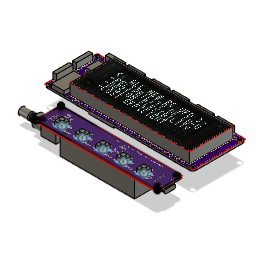
Overly Detailed Board Mockup (Autodesk Fusion 360 design; units mm, degrees)
Autodesk Fusion 360 part; units mm, degrees
sketch "Sketch1" plane through (0, 0, 0) normal (0, 1, 0) x (1, 0, 0)
  line L0 (0, 0) -> (24.384, 0)
  line L1 (24.384, 0) -> (24.384, 39.37)
  line L2 (24.384, 39.37) -> (0, 39.37)
  line L3 (0, 39.37) -> (0, 0)
  line L4 (7.1557, 6.35) -> (17.3157, 6.35)
  line L5 (17.3157, 6.35) -> (17.3157, 3.048)
  line L6 (17.3157, 3.048) -> (7.1557, 3.048)
  line L7 (7.1557, 3.048) -> (7.1557, 6.35)
  line L8 (7.1557, 6.35) -> (17.3157, 3.048) construction
  line L9 (17.3157, 6.35) -> (7.1557, 3.048) construction
  point P0 (12.2357, 4.699)
  dimension "d1" = 24.384
  dimension "d2" = 39.37
  dimension "d3" = 3.302
  dimension "d4" = 10.16
  dimension "d6" = 33.02
  constraint horizontal L0
  constraint vertical L1
  constraint horizontal L2
  constraint vertical L3
  constraint coincident L0.start L3.end
  constraint perpendicular L4 L5
  constraint parallel L4 L6
  constraint parallel L5 L7
  constraint horizontal L4
  constraint coincident L8 P0
  constraint coincident L9 P0
  measures "d1" distance of L0.start L0.end
  measures "d2" distance of L0.start L2.end
  measures "d3" distance of L4.end L5.end
  measures "d4" distance of L5.end L6.end
  measures "d6" distance of L2 L4
extrude "Extrude1" add sketch "Sketch1" along normal blind 1.905 contours L0 L1 L2 L3 | L4 L5 L6 L7 makes body 1
extrude "Extrude2" cut sketch "Sketch1" along normal through all contours L4 L5 L6 L7 bodies 1
sketch "Sketch2" plane through (0, 0, 0) normal (0, -1, 0) x (1, 0, 0)
  line L0 (17.3157, -3.048) -> (17.3157, -6.35)
  line L1 (17.3157, -6.35) -> (7.1557, -6.35)
  line L2 (7.1557, -6.35) -> (7.1557, -3.048)
  line L3 (7.1557, -3.048) -> (17.3157, -3.048)
  line L4 (0, 0) -> (0, -39.37)
  line L5 (0, -39.37) -> (24.384, -39.37)
  line L6 (24.384, -39.37) -> (24.384, 0)
  line L7 (24.384, 0) -> (0, 0)
  line L8 (-3.683, -39.37) -> (-2.54, -19.9644)
  line L9 (-2.54, -19.9644) -> (-1.8129, -7.62)
  line L10 (26.924, -19.9644) -> (26.1969, -7.62)
  line L11 (28.067, -39.37) -> (26.924, -19.9644)
  line L12 (-1.8129, -7.62) -> (26.1969, -7.62)
  line L13 (28.067, -39.37) -> (-3.683, -39.37)
  dimension "d15" = 93.371
  dimension "d16" = 93.371
  dimension "d17" = 31.75
  dimension "d18" = 31.75
  constraint parallel L8 L9
  constraint parallel L10 L11
  constraint horizontal L12
  constraint perpendicular L4 L13
  measures "d15" angle of L11 L13
  measures "d16" angle of L8 L13
  measures "d17" horizontal distance of L8.start L11.start
  measures "d18" distance of L12 L13
extrude "Extrude3" add sketch "Sketch2" along normal blind 3.175 contours L4 L5 L6 L12 L13 | L4 L8 L9 L12 L13 | L6 L10 L11 L12 L13 bodies 1
sketch "Sketch3" plane through (0, 0, -39.37) normal (0, 0, -1) x (-1, 0, 0)
  line L0 (0, 0) -> (0, 1.905)
  line L1 (0, 1.905) -> (-24.384, 1.905)
  line L2 (-24.384, 1.905) -> (-24.384, 0)
  line L3 (-24.384, 0) -> (-28.067, 0)
  line L4 (-28.067, 0) -> (-28.067, -3.175)
  line L5 (-28.067, -3.175) -> (3.683, -3.175)
  line L6 (3.683, -3.175) -> (3.683, 0)
  line L7 (3.683, 0) -> (0, 0)
  line L8 (-24.384, 0) -> (-28.067, -0.762)
  line L9 (0, 0) -> (3.683, -0.762)
  dimension "d21" = 0.762
  dimension "d22" = 0.762
  constraint coincident L2.end L3.start
  constraint coincident L4 L8.end
  constraint coincident L0.start L7.end
  constraint coincident L6 L9.end
  measures "d21" distance of L3.end L8.end
  measures "d22" distance of L6.end L9.end
extrude "Extrude4" cut sketch "Sketch3" against normal through all contours L0 L1 L2 L4 L5 L6 L8 L9 keep common part bodies 1
sketch "Sketch4" plane through (24.384, 0, 0) normal (1, 0, 0) x (0, 0, -1)
  line L0 (0, 0) -> (7.62, 0)
  line L1 (7.62, 0) -> (39.37, 0)
  line L2 (39.37, 0) -> (39.37, 1.905)
  line L3 (39.37, 1.905) -> (0, 1.905)
  line L4 (0, 1.905) -> (0, 0)
  line L5 (0, 1.905) -> (3.048, 0)
  line L6 (3.048, 0) -> (0, 0)
  line L7 (0, 1.905) -> (0, 0)
  point P0 (3.048, 0)
  constraint coincident L3.end L4.start
  constraint coincident P0 L5.end
  constraint coincident L0.start L4.end
extrude "Extrude5" cut sketch "Sketch4" against normal through all contours L0 L4 L5 L6 L7 bodies 1
sketch "Sketch5" plane through (0, 0, 0) normal (0, 1, 0) x (1, 0, 0)
  line L0 (2.54, 0) -> (116.84, 0)
  line L1 (119.38, 2.54) -> (119.38, 40.132)
  line L2 (116.84, 42.672) -> (2.54, 42.672)
  line L3 (0, 40.132) -> (0, 2.54)
  arc A0 (2.54, 42.672) -> (0, 40.132) centre (2.54, 40.132) ccw
  arc A1 (0, 2.54) -> (2.54, 0) centre (2.54, 2.54) ccw
  arc A2 (116.84, 0) -> (119.38, 2.54) centre (116.84, 2.54) ccw
  arc A3 (119.38, 40.132) -> (116.84, 42.672) centre (116.84, 40.132) ccw
  circle A4 centre (2.54, 40.132) radius 1.4132
  circle A5 centre (116.84, 40.132) radius 1.4368
  circle A6 centre (116.8086, 2.6914) radius 1.4384
  circle A7 centre (2.54, 2.6919) radius 1.4095
  point P0 (119.38, 0)
  point P1 (0, 42.672)
  dimension "d25" = 42.672
  dimension "d26" = 119.38
  dimension "d27" = 2.54
  dimension "d28" = 2.54
  dimension "d29" = 2.54
  dimension "d30" = 2.54
  constraint horizontal L0
  constraint vertical L1
  constraint horizontal L2
  constraint vertical L3
  constraint coincident P1 L2
  constraint coincident P1 L3
  constraint tangent L2 A0
  constraint tangent L3 A0
  constraint coincident origin L0
  constraint coincident origin L3
  constraint tangent L0 A1
  constraint tangent L3 A1
  constraint coincident P0 L1
  constraint coincident P0 L0
  constraint tangent L1 A2
  constraint tangent L0 A2
  constraint tangent L2 A3
  constraint tangent L1 A3
  constraint concentric A0 A4
  constraint concentric A3 A5
  measures "d25" distance of origin P1
  measures "d26" distance of origin P0
  measures "d27" radius of A0
  measures "d28" radius of A1
  measures "d29" radius of A2
  measures "d30" radius of A3
extrude "Extrude6" add sketch "Sketch5" against normal blind 1.6256 separate body makes body 2
sketch "Sketch6" plane through (0, 0, 0) normal (0, 1, 0) x (-1, 0, 0)
  circle A0 centre (-2.54, -2.6919) radius 1.4095
  circle A1 centre (-116.8086, -2.6914) radius 1.4384
  circle A2 centre (-2.54, -40.132) radius 1.4132
  circle A3 centre (-116.84, -40.132) radius 1.4368
  arc A4 (-119.38, -40.132) -> (-116.84, -42.672) centre (-116.84, -40.132) ccw
  line L0 (-116.84, -42.672) -> (-2.54, -42.672)
  arc A5 (-2.54, -42.672) -> (0, -40.132) centre (-2.54, -40.132) ccw
  line L1 (0, -40.132) -> (0, -2.54)
  arc A6 (0, -2.54) -> (-2.54, 0) centre (-2.54, -2.54) ccw
  line L2 (-2.54, 0) -> (-116.84, 0)
  arc A7 (-116.84, 0) -> (-119.38, -2.54) centre (-116.84, -2.54) ccw
  line L3 (-119.38, -2.54) -> (-119.38, -40.132)
  line L4 (-18.034, -2.667) -> (-113.9534, -2.667)
  line L5 (-113.9534, -2.667) -> (-113.9534, -37.5746)
  line L6 (-113.9534, -37.5746) -> (-18.034, -37.5746)
  line L7 (-18.034, -37.5746) -> (-18.034, -2.667)
  line L8 (-3.048, -6.858) -> (0, -6.858)
  line L9 (0, -6.858) -> (0, -20.066)
  line L10 (0, -20.066) -> (-3.048, -20.066)
  line L11 (-3.048, -20.066) -> (-3.048, -6.858)
  line L12 (-3.048, -22.7169) -> (0, -22.7169)
  line L13 (0, -22.7169) -> (0, -35.9458)
  line L14 (0, -35.9458) -> (-3.048, -35.9458)
  line L15 (-3.048, -35.9458) -> (-3.048, -22.7169)
  line L16 (-9.5782, -39.5447) -> (-22.7925, -39.5447)
  line L17 (-22.7925, -39.5447) -> (-22.7925, -42.672)
  line L18 (-22.7925, -42.672) -> (-9.5782, -42.672)
  line L19 (-9.5782, -42.672) -> (-9.5782, -39.5447)
  line L20 (-25.4303, -39.5447) -> (-38.6971, -39.5447)
  line L21 (-38.6971, -39.5447) -> (-38.6971, -42.672)
  line L22 (-38.6971, -42.672) -> (-25.4303, -42.672)
  line L23 (-25.4303, -42.672) -> (-25.4303, -39.5447)
  line L24 (-45.085, -39.624) -> (-58.3441, -39.624)
  line L25 (-58.3441, -39.624) -> (-58.3441, -42.672)
  line L26 (-58.3441, -42.672) -> (-45.085, -42.672)
  line L27 (-45.085, -42.672) -> (-45.085, -39.624)
  line L28 (-60.957, -39.5595) -> (-74.2397, -39.5595)
  line L29 (-74.2397, -39.5595) -> (-74.2397, -42.672)
  line L30 (-74.2397, -42.672) -> (-60.957, -42.672)
  line L31 (-60.957, -42.672) -> (-60.957, -39.5595)
  line L32 (-80.7977, -39.5595) -> (-94.107, -39.5595)
  line L33 (-94.107, -39.5595) -> (-94.107, -42.672)
  line L34 (-94.107, -42.672) -> (-80.7977, -42.672)
  line L35 (-80.7977, -42.672) -> (-80.7977, -39.5595)
  line L36 (-97.0058, -39.5595) -> (-110.2962, -39.5595)
  line L37 (-110.2962, -39.5595) -> (-110.2962, -42.672)
  line L38 (-110.2962, -42.672) -> (-97.0058, -42.672)
  line L39 (-97.0058, -42.672) -> (-97.0058, -39.5595)
  line L40 (-5.8246, -17.9754) -> (-15.8155, -17.9754)
  line L41 (-15.8155, -17.9754) -> (-15.8155, -0.0082)
  line L42 (-15.8155, -0.0082) -> (-5.8246, -0.0082)
  line L43 (-5.8246, -0.0082) -> (-5.8246, -17.9754)
  line L44 (-6.9981, -36.3389) -> (-17.116, -36.3389)
  line L45 (-17.116, -36.3389) -> (-17.116, -26.105)
  line L46 (-17.116, -26.105) -> (-6.9981, -26.105)
  line L47 (-6.9981, -26.105) -> (-6.9981, -36.3389)
  constraint horizontal L4
  constraint vertical L5
  constraint horizontal L6
  constraint vertical L7
  constraint horizontal L8
  constraint vertical L9
  constraint horizontal L10
  constraint vertical L11
  constraint coincident L1 L9.end
  constraint horizontal L12
  constraint vertical L13
  constraint horizontal L14
  constraint vertical L15
  constraint coincident L1 L13.end
  constraint horizontal L16
  constraint vertical L17
  constraint horizontal L18
  constraint vertical L19
  constraint coincident L0 L17.end
  constraint horizontal L20
  constraint vertical L21
  constraint horizontal L22
  constraint vertical L23
  constraint coincident L0 L21.end
  constraint horizontal L24
  constraint vertical L25
  constraint horizontal L26
  constraint vertical L27
  constraint coincident L0 L25.end
  constraint horizontal L28
  constraint vertical L29
  constraint horizontal L30
  constraint vertical L31
  constraint coincident L0 L29.end
  constraint horizontal L32
  constraint vertical L33
  constraint horizontal L34
  constraint vertical L35
  constraint coincident L0 L33.end
  constraint horizontal L36
  constraint vertical L37
  constraint horizontal L38
  constraint vertical L39
  constraint coincident L0 L37.end
  constraint horizontal L40
  constraint vertical L41
  constraint horizontal L42
  constraint vertical L43
  constraint horizontal L44
  constraint vertical L45
  constraint horizontal L46
  constraint vertical L47
extrude "Extrude8" add sketch "Sketch6" along normal blind 8.5 separate body contours L4 L5 L6 L7 makes body 3
extrude "Extrude9" add sketch "Sketch6" along normal blind 5 separate body contours L0 L36 L37 L38 L39 | L0 L32 L33 L34 L35 | L1 L8 L9 L10 L11 | L0 L28 L29 L30 L31 | L1 L12 L13 L14 L15 | L0 L24 L25 L26 L27 | L0 L20 L21 L22 L23 | L0 L16 L17 L18 L19 makes body 4 at (65.3846, 1.6667, -39.5595) makes body 5 at (0, 1.6667, -15.6633) makes body 6 at (18.3877, 1.6667, -42.672) makes body 7 at (85.2341, 1.6667, -39.5595) makes body 8 at (49.5047, 1.6667, -39.624) makes body 9 at (0, 1.6667, -31.5362) makes body 10 at (29.8526, 1.6667, -39.5447) makes body 11 at (101.4359, 1.6667, -39.5595)
combine "Combine1" operation add target body 2 tool bodies 11 3 4 5 6 8 7 10 9
extrude "Extrude10" add sketch "Sketch6" along normal blind 3.2 contours L40 L41 L42 L43 bodies 2
extrude "Extrude11" add sketch "Sketch6" along normal blind 2.1 contours L44 L45 L46 L47 bodies 2
copy_body "Body->Comp1" bodies 2 removing the originals makes body 12 in component "Mainboard Mockup"
sketch "Sketch7" plane through (0, -1.6256, 0) normal (0, -1, 0) x (1, 0, 0)
  circle A0 centre (2.54, -2.6919) radius 1.4095
  circle A1 centre (116.8086, -2.6914) radius 1.4384
  circle A2 centre (2.54, -40.132) radius 1.4132
  circle A3 centre (116.84, -40.132) radius 1.4368
  arc A4 (116.84, -42.672) -> (119.38, -40.132) centre (116.84, -40.132) ccw
  line L0 (119.38, -40.132) -> (119.38, -2.54)
  arc A5 (119.38, -2.54) -> (116.84, 0) centre (116.84, -2.54) ccw
  line L1 (116.84, 0) -> (2.54, 0)
  arc A6 (2.54, 0) -> (0, -2.54) centre (2.54, -2.54) ccw
  line L2 (0, -2.54) -> (0, -40.132)
  arc A7 (0, -40.132) -> (2.54, -42.672) centre (2.54, -40.132) ccw
  line L3 (2.54, -42.672) -> (116.84, -42.672)
  line L4 (56.9773, -8.2444) -> (34.4218, -8.2444)
  line L5 (34.4218, -8.2444) -> (34.4218, -13.7635)
  line L6 (34.4218, -13.7635) -> (56.9773, -13.7635)
  line L7 (56.9773, -13.7635) -> (56.9773, -8.2444)
  line L8 (55.7007, -8.2444) -> (35.814, -8.2444)
  line L9 (35.814, -8.2444) -> (35.814, 0)
  line L10 (35.814, 0) -> (55.7007, 0)
  line L11 (55.7007, 0) -> (55.7007, -8.2444)
  line L12 (109.728, -3.302) -> (74.168, -3.302)
  line L13 (74.168, -3.302) -> (74.168, -1.778)
  line L14 (74.168, -1.778) -> (109.728, -1.778)
  line L15 (109.728, -1.778) -> (109.728, -3.302)
  line L16 (29.21, -3.302) -> (23.622, -3.302)
  line L17 (23.622, -3.302) -> (23.622, -1.778)
  line L18 (23.622, -1.778) -> (29.21, -1.778)
  line L19 (29.21, -1.778) -> (29.21, -3.302)
  circle A8 centre (103.2884, -11.0072) radius 4.825
  constraint horizontal L4
  constraint vertical L5
  constraint horizontal L6
  constraint vertical L7
  constraint horizontal L8
  constraint vertical L9
  constraint horizontal L10
  constraint vertical L11
  constraint coincident L1 L9.end
  constraint coincident L4 L8.start
  constraint horizontal L12
  constraint vertical L13
  constraint horizontal L14
  constraint vertical L15
  constraint horizontal L16
  constraint vertical L17
  constraint horizontal L18
  constraint vertical L19
extrude "Extrude1'" add sketch "Sketch7" along normal blind 1.905 contours L1 L4 L8 L9 L10 L11 | L12 L13 L14 L15 | L16 L17 L18 L19 bodies 12 in component "Mainboard Mockup"
extrude "Extrude2'" add sketch "Sketch7" along normal blind 2 contours L4 L5 L6 L7 L8 bodies 12 in component "Mainboard Mockup"
extrude "Extrude3'" add sketch "Sketch7" along normal blind 3 contours A8 bodies 12 in component "Mainboard Mockup"
extrude "Extrude4'" cut 1 faces at (49.0718, -3.5306, -5.4963) along direction (0, 1, 0) blind 0.635 on bodies 12 bodies 12 in component "Mainboard Mockup"
sketch "Sketch1 (2)" plane through (0, 0, 0) normal (0, 1, 0) x (1, 0, 0) in component "Control Board Mockup"
  line L0 (2.54, 0) -> (95.25, 0)
  line L1 (97.79, 2.54) -> (97.79, 17.78)
  line L2 (95.25, 20.32) -> (2.54, 20.32)
  line L3 (0, 17.78) -> (0, 2.54)
  arc A0 (2.54, 20.32) -> (0, 17.78) centre (2.54, 17.78) ccw
  arc A1 (0, 2.54) -> (2.54, 0) centre (2.54, 2.54) ccw
  arc A2 (97.79, 17.78) -> (95.25, 20.32) centre (95.25, 17.78) ccw
  arc A3 (95.25, 0) -> (97.79, 2.54) centre (95.25, 2.54) ccw
  line L4 (11.7174, 3.3756) -> (17.6784, 3.3756)
  line L5 (17.6784, 3.3756) -> (17.6784, 9.3472)
  line L6 (17.6784, 9.3472) -> (11.7174, 9.3472)
  line L7 (11.7174, 9.3472) -> (11.7174, 3.3756)
  circle A4 centre (14.732, 6.35) radius 1.7145
  circle A5 centre (31.1912, 6.35) radius 1.7145
  line L8 (28.1766, 9.3472) -> (28.1766, 3.3756)
  line L9 (34.1376, 9.3472) -> (28.1766, 9.3472)
  line L10 (28.1766, 3.3756) -> (34.1376, 3.3756)
  line L11 (34.1376, 3.3756) -> (34.1376, 9.3472)
  circle A6 centre (47.6504, 6.35) radius 1.7145
  line L12 (44.6358, 9.3472) -> (44.6358, 3.3756)
  line L13 (50.5968, 9.3472) -> (44.6358, 9.3472)
  line L14 (44.6358, 3.3756) -> (50.5968, 3.3756)
  line L15 (50.5968, 3.3756) -> (50.5968, 9.3472)
  circle A7 centre (64.1096, 6.35) radius 1.7145
  line L16 (61.095, 9.3472) -> (61.095, 3.3756)
  line L17 (67.056, 9.3472) -> (61.095, 9.3472)
  line L18 (61.095, 3.3756) -> (67.056, 3.3756)
  line L19 (67.056, 3.3756) -> (67.056, 9.3472)
  circle A8 centre (80.5688, 6.35) radius 1.7145
  line L20 (77.5542, 9.3472) -> (77.5542, 3.3756)
  line L21 (83.5152, 9.3472) -> (77.5542, 9.3472)
  line L22 (77.5542, 3.3756) -> (83.5152, 3.3756)
  line L23 (83.5152, 3.3756) -> (83.5152, 9.3472)
  point P0 (97.79, 0)
  point P1 (0, 20.32)
  dimension "d51" = 97.79
  dimension "d52" = 20.32
  dimension "d53" = 2.54
  dimension "d54" = 2.54
  dimension "d55" = 2.54
  dimension "d56" = 2.54
  dimension "d57" = 3.429
  dimension "d60" = 16.4592
  dimension "d61" = 0
  constraint horizontal L0
  constraint vertical L1
  constraint horizontal L2
  constraint vertical L3
  constraint coincident P1 L2
  constraint coincident P1 L3
  constraint tangent L2 A0
  constraint tangent L3 A0
  constraint coincident origin L0
  constraint coincident origin L3
  constraint tangent L0 A1
  constraint tangent L3 A1
  constraint tangent L2 A2
  constraint tangent L1 A2
  constraint coincident P0 L1
  constraint coincident P0 L0
  constraint tangent L1 A3
  constraint tangent L0 A3
  constraint horizontal L4
  constraint vertical L5
  constraint horizontal L6
  constraint vertical L7
  measures "d51" distance of origin P0
  measures "d52" distance of origin P1
  measures "d53" radius of A0
  measures "d54" radius of A1
  measures "d55" radius of A2
  measures "d56" radius of A3
  measures "d57" diameter of A4
extrude "Extrude1''" add sketch "Sketch1 (2)" against normal blind 1.6256 separate body contours L0 L1 L2 L3 A0 A1 A2 A3 | L4 L5 L6 L7 | A4 | A5 | L8 L9 L10 L11 | A6 | L12 L13 L14 L15 | A7 | L16 L17 L18 L19 | A8 | L20 L21 L22 L23 makes body 13 in component "Control Board Mockup"
extrude "Extrude2''" add sketch "Sketch1 (2)" along normal blind 3.81 contours L4 L5 L6 L7 | L8 L9 L10 L11 | L12 L13 L14 L15 | L16 L17 L18 L19 | L20 L21 L22 L23 bodies 13 in component "Control Board Mockup"
extrude "Extrude3''" add sketch "Sketch1 (2)" along normal blind 5.0038 contours A4 | A5 | A6 | A7 | A8 bodies 13 in component "Control Board Mockup"
sketch "Sketch2 (2)" plane through (0, -1.6256, 0) normal (0, -1, 0) x (1, 0, 0) in component "Control Board Mockup"
  arc A0 (97.79, -2.54) -> (95.25, 0) centre (95.25, -2.54) ccw
  line L0 (95.25, 0) -> (2.54, 0)
  arc A1 (2.54, 0) -> (0, -2.54) centre (2.54, -2.54) ccw
  line L1 (0, -2.54) -> (0, -17.78)
  arc A2 (0, -17.78) -> (2.54, -20.32) centre (2.54, -17.78) ccw
  line L2 (2.54, -20.32) -> (95.25, -20.32)
  arc A3 (95.25, -20.32) -> (97.79, -17.78) centre (95.25, -17.78) ccw
  line L3 (97.79, -17.78) -> (97.79, -2.54)
  line L4 (12.0798, -13.738) -> (0, -13.738)
  line L5 (0, -13.738) -> (0, -4.064)
  line L6 (0, -4.064) -> (12.0798, -4.064)
  line L7 (12.0798, -4.064) -> (12.0798, -13.738)
  line L8 (18.3553, -1.1964) -> (78.1042, -1.1964)
  line L9 (78.1042, -1.1964) -> (78.1042, -16.6847)
  line L10 (78.1042, -16.6847) -> (18.3553, -16.6847)
  line L11 (18.3553, -16.6847) -> (18.3553, -1.1964)
  line L12 (88.2501, -13.6825) -> (98.7501, -13.6825)
  line L13 (98.7501, -13.6825) -> (98.7501, -4.4825)
  line L14 (98.7501, -4.4825) -> (88.2501, -4.4825)
  line L15 (88.2501, -4.4825) -> (88.2501, -13.6825)
  dimension "d68" = 10.5
  dimension "d69" = 9.2
  constraint horizontal L4
  constraint vertical L5
  constraint horizontal L6
  constraint vertical L7
  constraint coincident L1 L5.end
  constraint horizontal L8
  constraint vertical L9
  constraint horizontal L10
  constraint vertical L11
  constraint horizontal L12
  constraint vertical L13
  constraint horizontal L14
  constraint vertical L15
  measures "d68" distance of L12.start L12.end
  measures "d69" distance of L12.start L14.end
extrude "Extrude4''" add sketch "Sketch2 (2)" along normal blind 14.859 contours L8 L9 L10 L11 bodies 13 in component "Control Board Mockup"
extrude "Extrude5'" add sketch "Sketch2 (2)" along normal blind 3.28 contours L3 L12 L13 L14 | L3 L12 L14 L15 bodies 13 in component "Control Board Mockup"
extrude "Extrude6'" add sketch "Sketch2 (2)" along normal blind 11.3538 contours L1 L4 L5 L6 L7 bodies 13 in component "Control Board Mockup"
sketch "Sketch3 (2)" plane through (0, 0, 0) normal (0, 0, 1) x (1, 0, 0) in component "Control Board Mockup"
  line L0 (0, -1.6256) -> (0, -12.9794)
  line L1 (0, -6.477) -> (-20, -6.477)
  line L2 (0, -12.9794) -> (12.0798, -12.9794)
  line L3 (0, -11.43) -> (-7, -11.43)
  line L4 (-7, -11.43) -> (-7, -8.3975)
  line L5 (-7, -8.3975) -> (-9.5, -8.3975)
  line L6 (-9.5, -8.3975) -> (-9.5, -9.477)
  line L7 (-9.5, -9.477) -> (-10.3561, -9.477)
  line L8 (-10.3561, -9.477) -> (-11, -8.8331)
  line L9 (-11, -8.8331) -> (-12, -8.8331)
  line L10 (-12, -8.8331) -> (-12.6439, -9.477)
  line L11 (-12.6439, -9.477) -> (-20, -9.477)
  line L12 (-20, -9.477) -> (-20, -6.477)
  line L13 (0, -11.43) -> (0, -6.477)
  dimension "d76" = 20
  dimension "d77" = 6.5024
  dimension "d78" = 135
  dimension "d80" = 135
  dimension "d82" = 7
  dimension "d85" = 8
  dimension "d86" = 9
  dimension "d87" = 2.5
  dimension "d88" = 3
  constraint coincident L0 L1.start
  constraint coincident L0 L3.start
  constraint perpendicular L0 L3
  constraint perpendicular L3 L4
  constraint perpendicular L4 L5
  constraint perpendicular L5 L6
  constraint perpendicular L6 L7
  constraint horizontal L9
  constraint parallel L1 L11
  constraint perpendicular L1 L12
  constraint collinear L7 L11
  measures "d76" distance of L1.start L1.end
  measures "d77" distance of L1 L2
  measures "d78" angle of L7 L8
  measures "d80" angle of L9 L10
  measures "d82" horizontal distance of L3.start L3.end
  measures "d85" distance of L9.end L12
  measures "d86" distance of L8.end L12
  measures "d87" horizontal distance of L4.end L5.end
  measures "d88" vertical distance of L1.end L11.end
revolve "Revolve1" add sketch "Sketch3 (2)" angle 360 about axis through (0, -6.477, 0) along (-1, 0, 0) separate body makes body 14 in component "Control Board Mockup"
move_body "Move1" bodies 14 to x (1, 0, 0) y (0, 1, 0) z (0, 0, 1) at (0, -1.5494, -8.901) in component "Control Board Mockup"
fillet "Fillet1" radius 1.524 4 edges at (98.27, -1.6256, -4.4825) (93.5001, -4.9056, -4.4825) (93.5001, -4.9056, -13.6825) (98.27, -1.6256, -13.6825) on bodies 13 in component "Control Board Mockup"
component "Mainboard Mockup" placed x (1, 0, 0) y (0, 1, 0) z (0, 0, 1) at (0, 0, 0)
component "Control Board Mockup" placed x (1, 0, 0) y (0, 1, 0) z (0, 0, 1) at (0, 0, 0)
hidden bodies 1
equation "d74 = 0.191 in + 0.256 in"
